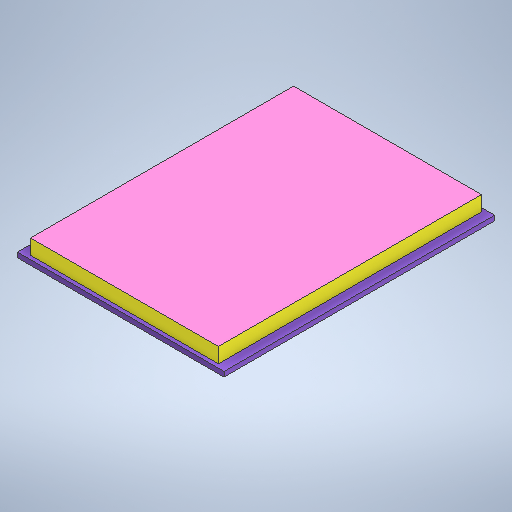
# Autodesk Inventor part: display
Saved by Autodesk Inventor 2025.2 (Build 292293000, 293)
## iProperties
Created: 2025-08-16
Part Number: display
Material: Generic
Document SubType Name: Modeling
Designer: pakiyan
Density: 1 g/cm^3
Appearance: Default
Author: pakiyan
Autodesk Inventor part; units mm, degrees
ref_plane "YZ Plane" through (0, 0, 0) normal (1, 0, 0) x (0, 1, 0)
ref_plane "XZ Plane" through (0, 0, 0) normal (0, 1, 0) x (-1, 0, 0)
ref_plane "XY Plane" through (0, 0, 0) normal (0, 0, 1) x (1, 0, 0)
sketch "Sketch1" plane through (0, 0, 0) normal (0, 1, 0) x (-1, 0, 0)
  line L0 (27.5, 36) -> (-27.5, 36)
  line L1 (-27.5, 36) -> (-27.5, -36)
  line L2 (-27.5, -36) -> (27.5, -36)
  line L3 (27.5, -36) -> (27.5, 36)
  line L4 (27.5, 36) -> (-27.5, -36) construction
  line L5 (-27.5, 36) -> (27.5, -36) construction
  point P0 (0, 0)
  dimension "d0" = 55
  dimension "d1" = 72
  constraints: 12 end point, 2 midpoint, 2 parallel, 1 horizontal, 1 perpendicular
  measures "d0" distance of L0.start L0.end
  measures "d1" distance of L2.end L0.start
extrude "Extrusion1" add sketch "Sketch1" along normal blind 1.3
sketch "Sketch2" plane through (0, 1.3, 0) normal (0, 1, 0) x (1, 0, 0)
  line L0 (-25, 35) -> (25, 35)
  line L1 (25, 35) -> (25, -35)
  line L2 (25, -35) -> (-25, -35)
  line L3 (-25, -35) -> (-25, 35)
  line L4 (-25, 35) -> (25, -35) construction
  line L5 (25, 35) -> (-25, -35) construction
  point P0 (0, 0)
  dimension "d4" = 70
  dimension "d5" = 50
  constraints: 12 end point, 2 midpoint, 2 parallel, 1 horizontal, 1 perpendicular
  measures "d4" distance of L0.end L1.end
  measures "d5" distance of L1.end L2.end
extrude "Extrusion2" add sketch "Sketch2" along normal blind 4
sketch "Sketch3" plane through (0, 0, 0) normal (0, -1, 0) x (1, 0, 0)
  line L0 (-27.5, -17) -> (-22.5, -17)
  line L1 (-22.5, -17) -> (-22.5, 13)
  line L2 (-22.5, 13) -> (-27.5, 13)
  line L3 (-27.5, 13) -> (-27.5, -17)
  line L4 (27.5, -36) -> (-27.5, -36) projected
  line L5 (-27.5, -36) -> (-27.5, 36) projected
  point P0 (0, 0)
  dimension "d8" = 30
  dimension "d9" = 5
  dimension "d10" = 19
  dimension "d11" = 0
  constraints: 8 end point, 2 parallel, 1 horizontal, 1 perpendicular
  measures "d8" distance of L2.end L0.start
  measures "d9" distance of L0.start L0.end
  measures "d10" distance between parallel lines of L4 L0
  measures "d11" distance between parallel lines of L5 L3
extrude "Extrusion3" add sketch "Sketch3" along normal blind 13
body "Solid1"
